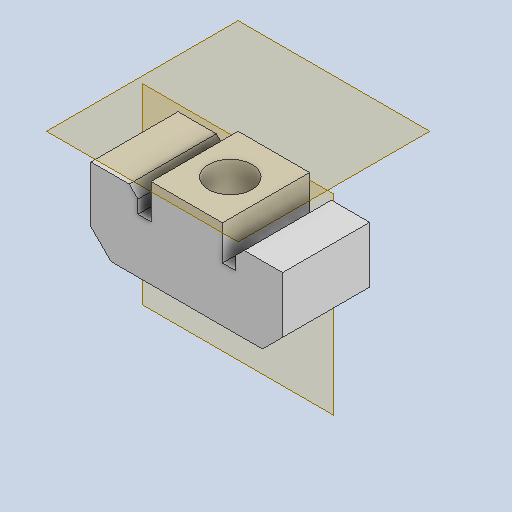
# Autodesk Inventor part: Pecinha do perfil_CPY
Saved by Autodesk Inventor 2024 (Build 280153000, 153)
## iProperties
Created: 2024-05-05
Part Number: Pecinha do perfil_CPY
Material: Alumínio
Document SubType Name: Modeling
Designer: mathe
Density: 2.7 g/cm^3
Appearance: Padrão
Title: perfil_40x40_200 v2.step
Sending System: Autodesk Translation Framework v12.20.1.177
Preprocessor: ST-DEVELOPER v20
Autodesk Inventor part; units mm, degrees
ref_plane "YZ Plane" through (0, 0, 0) normal (1, 0, 0) x (0, 1, 0)
ref_plane "XZ Plane" through (0, 0, 0) normal (0, 1, 0) x (-1, 0, 0)
ref_plane "XY Plane" through (0, 0, 0) normal (0, 0, 1) x (1, 0, 0)
ref_plane "Plano de trabalho2" through (-4.1, 8.25, 200) normal (0, 0, 1) x (1, 0, 0)
sketch "Esboço2" plane through (-4.1, 8.25, 200) normal (0, 0, 1) x (1, 0, 0)
  line L0 (-6.9, 3.8107) -> (-6.9, 10.25) projected
  line L1 (-6.9, 10.25) -> (-6.9, 3.8107)
  line L2 (12.7893, 1.5) -> (-4.5893, 1.5) projected
  line L3 (-6.9, 3.8107) -> (-4.5893, 1.5)
  line L4 (-4.5893, 1.5) -> (12.7893, 1.5)
  line L5 (12.7893, 1.5) -> (15.1, 3.8107)
  line L6 (15.1, 10.25) -> (15.1, 3.8107) projected
  line L7 (15.1, 3.8107) -> (15.1, 10.25)
  line L8 (10.7, 10.25) -> (15.1, 10.25) projected
  line L9 (15.1, 10.25) -> (10.7, 10.25)
  line L10 (9.7, 7.75) -> (9.7, 9.25) projected
  line L11 (10.7, 10.25) -> (9.7, 9.25)
  line L12 (9.7, 9.25) -> (9.7, 7.75)
  line L13 (9.7, 7.75) -> (8.2, 7.75)
  line L14 (15.1, 11.75) -> (8.2, 11.75) projected
  line L15 (8.2, 7.75) -> (8.2, 11.75)
  line L16 (0, 7.75) -> (0, 11.75) projected
  line L17 (8.2, 11.75) -> (0, 11.75)
  line L18 (0, 11.75) -> (0, 7.75)
  line L19 (0, 7.75) -> (-1.5, 7.75)
  line L20 (-2.5, 10.25) -> (-1.5, 9.25) projected
  line L21 (-1.5, 7.75) -> (-1.5, 9.25)
  line L22 (-1.5, 9.25) -> (-2.5, 10.25)
  line L23 (-2.5, 10.25) -> (-6.9, 10.25)
  point P0 (4.1, -8.25)
  constraints: 32 end point, 7 perpendicular, 5 collinear, 3 point on line, 2 parallel
extrude "Extrusão1" add sketch "Esboço2" along normal blind 10
ref_plane "Plano de trabalho5" through (-4.1, 20, 200) normal (0, 1, 0) x (1, 0, 0)
sketch "Esboço3" plane through (-4.1, 20, 200) normal (0, 1, 0) x (1, 0, 0)
  circle A0 centre (4.1, -5) radius 2.5
  line L0 (19.5, 0) -> (-11.3, 0) projected
  line L1 (15.1, 0) -> (15.1, -10) projected
  point P0 (4.1, 200)
  dimension "d2" = 5
  dimension "d3" = 5
  dimension "d4" = 11
  constraints: 1 centre point
  measures "d2" diameter of A0
  measures "d3" distance from line of L0 A0.centre
  measures "d4" distance from line of L1 A0.centre
hole "Furo1" at (0, 20, 205) direction (0, -1, 0) diameter 5 depth 20 tip angle 118
